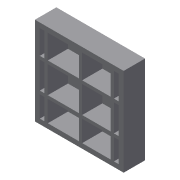
# Autodesk Inventor part: Toy Chassis
Saved by Autodesk Inventor 2015 (Build 190159000, 159)
## iProperties
Created: 2015-03-07
Part Number: Toy Chassis
Material: Generic
Document SubType Name: Modeling
Designer: Tanner
Density: 1 g/cm^3
Appearance: Default
Author: Tanner
Autodesk Inventor part; units mm, degrees
ref_plane "YZ Plane" through (0, 0, 0) normal (1, 0, 0) x (0, 1, 0)
ref_plane "XZ Plane" through (0, 0, 0) normal (0, 1, 0) x (-1, 0, 0)
ref_plane "XY Plane" through (0, 0, 0) normal (0, 0, 1) x (1, 0, 0)
sketch "Sketch1" plane through (0, 0, 0) normal (0, 0, 1) x (1, 0, 0)
  line L0 (0, 0) -> (55.4917, 0)
  line L1 (55.4917, 0) -> (55.4917, 55.1277)
  line L2 (55.4917, 55.1277) -> (0, 55.1277)
  line L3 (0, 55.1277) -> (0, 0)
  dimension "d0" = 55.4917
  dimension "d1" = 55.1277
  constraints: 8 end point, 2 parallel, 1 horizontal, 1 perpendicular
  measures "d0" distance of L2.end L1.end
  measures "d1" distance of L1.end L0.end
extrude "Extrusion1" add sketch "Sketch1" along normal blind 0.762
sketch "Sketch2" plane through (0, 0, 0.762) normal (0, 0, 1) x (1, 0, 0)
  line L0 (3.0388, 52.072) -> (52.4437, 52.072)
  line L1 (52.4437, 52.072) -> (52.4437, 3.048)
  line L2 (52.4437, 3.048) -> (3.0388, 3.048)
  line L3 (3.0388, 3.048) -> (3.0388, 52.072)
  line L4 (55.4917, 55.1277) -> (0, 55.1277) projected
  line L5 (55.4917, 0) -> (55.4917, 55.1277) projected
  line L6 (0, 55.1277) -> (0, 0) projected
  line L7 (0, 0) -> (55.4917, 0) projected
  dimension "d4" = 3.0557
  dimension "d5" = 3.048
  dimension "d6" = 3.0388
  dimension "d7" = 3.048
  constraints: 8 end point, 2 parallel, 1 horizontal, 1 perpendicular
  measures "d4" distance between parallel lines of L4 L0
  measures "d5" distance between parallel lines of L5 L1
  measures "d6" distance between parallel lines of L6 L3
  measures "d7" distance between parallel lines of L7 L2
extrude "Extrusion2" add sketch "Sketch2" along normal blind 12.6333
sketch "Sketch3" plane through (0, 0, 0.762) normal (0, 0, 1) x (1, 0, 0)
  line L0 (3.0388, 3.048) -> (3.0388, 52.072) projected
  line L1 (52.4437, 3.048) -> (52.4437, 52.072) projected
  line L2 (3.0388, 18.2516) -> (52.4437, 18.2516)
  line L3 (52.4437, 18.2516) -> (52.4437, 16.1969)
  line L4 (52.4437, 16.1969) -> (3.0388, 16.1969)
  line L5 (3.0388, 16.1969) -> (3.0388, 18.2516)
  line L6 (52.4437, 3.048) -> (3.0388, 3.048) projected
  line L7 (3.0388, 37.0686) -> (52.4437, 37.0686)
  line L8 (52.4437, 37.0686) -> (52.4437, 35.0112)
  line L9 (52.4437, 35.0112) -> (3.0388, 35.0112)
  line L10 (3.0388, 35.0112) -> (3.0388, 37.0686)
  line L11 (3.0388, 52.072) -> (52.4437, 52.072) projected
  line L12 (3.0388, 3.048) -> (52.4437, 3.048) projected
  line L13 (27.4802, 3.048) -> (29.5348, 3.048)
  line L14 (29.5348, 3.048) -> (29.5348, 52.072)
  line L15 (29.5348, 52.072) -> (27.4802, 52.072)
  line L16 (27.4802, 52.072) -> (27.4802, 3.048)
  line L17 (5.9731, 52.072) -> (8.0305, 52.072)
  line L18 (8.0305, 52.072) -> (8.0305, 3.048)
  line L19 (8.0305, 3.048) -> (5.9731, 3.048)
  line L20 (5.9731, 3.048) -> (5.9731, 52.072)
  line L21 (47.3023, 52.072) -> (49.3597, 52.072)
  line L22 (49.3597, 52.072) -> (49.3597, 3.048)
  line L23 (49.3597, 3.048) -> (47.3023, 3.048)
  line L24 (47.3023, 3.048) -> (47.3023, 52.072)
  point P0 (0, 0)
  dimension "d10" = 13.1489
  dimension "d11" = 2.0547
  dimension "d12" = 15.0034
  dimension "d13" = 2.0574
  dimension "d14" = 2.0547
  dimension "d15" = 24.4414
  dimension "d16" = 2.0574
  dimension "d17" = 2.9343
  dimension "d18" = 3.084
  dimension "d19" = 2.0574
  constraints: 40 end point, 10 parallel, 10 point on line, 5 horizontal, 5 perpendicular
  measures "d10" distance between parallel lines of L6 L4
  measures "d11" distance between parallel lines of L2 L4
  measures "d12" distance between parallel lines of L11 L7
  measures "d13" distance between parallel lines of L9 L7
  measures "d14" distance between parallel lines of L14 L16
  measures "d15" distance between parallel lines of L0 L16
  measures "d16" distance between parallel lines of L18 L20
  measures "d17" distance between parallel lines of L0 L20
  measures "d18" distance between parallel lines of L1 L22
  measures "d19" distance between parallel lines of L24 L22
extrude "Extrusion3" add sketch "Sketch3" along normal blind 12.6333 contours L0 L2 L20 L4 | L20 L4 L18 L6 | L20 L2 L18 L4 | L0 L7 L20 L9 | L20 L9 L18 L2 | L18 L2 L16 L4 | L16 L4 L14 L6 | L20 L7 L18 L9 | L16 L2 L14 L4 | L20 L11 L18 L7 | L18 L7 L16 L9 | L16 L9 L14 L2 | L14 L2 L24 L4 | L24 L4 L22 L6 | L16 L7 L14 L9 | L24 L2 L22 L4 | L16 L11 L14 L7 | L14 L7 L24 L9 | L24 L9 L22 L2 | L22 L2 L1 L4 | L24 L7 L22 L9 | L24 L11 L22 L7 | L22 L7 L1 L9
body "Solid1"
